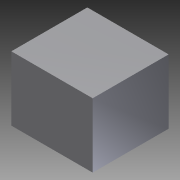
# Autodesk Inventor part: marc cube
Saved by Autodesk Inventor 2011 SP1 (Build 150282100, 282)
## iProperties
Created: 2013-01-14
Part Number: marc cube
Document SubType Name: Modeling
Designer: 355283
Density: 1 g/cm^3
Author: 355283
Autodesk Inventor part; units mm, degrees
ref_plane "YZ Plane" through (0, 0, 0) normal (1, 0, 0) x (0, 1, 0)
ref_plane "XZ Plane" through (0, 0, 0) normal (0, 1, 0) x (-1, 0, 0)
ref_plane "XY Plane" through (0, 0, 0) normal (0, 0, 1) x (1, 0, 0)
sketch "Sketch1" plane through (0, 0, 0) normal (0, 0, 1) x (1, 0, 0)
  line L0 (-11.1562, 7.6572) -> (16.0243, 7.6572)
  line L1 (16.0243, 7.6572) -> (16.0243, -13.8438)
  line L2 (16.0243, -13.8438) -> (-11.1562, -13.8438)
  line L3 (-11.1562, -13.8438) -> (-11.1562, 7.6572)
  point P0 (0, 0)
  constraints: 8 end point, 2 parallel, 1 horizontal, 1 perpendicular
extrude "Extrusion1" add sketch "Sketch1" along normal blind 25.4
body "Solid1"
